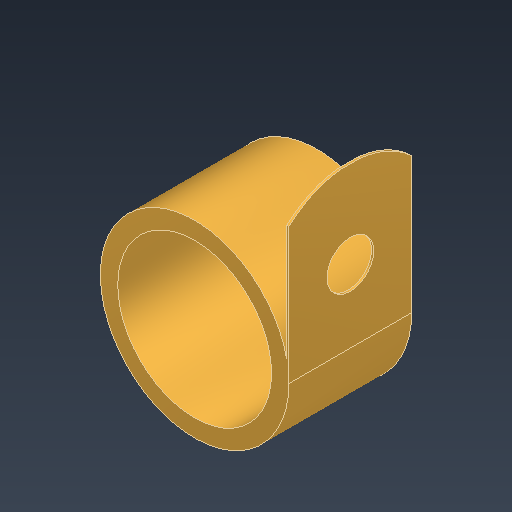
# Autodesk Inventor part: LCF 025 05 031S (on hub)
Saved by Autodesk Inventor 2021.3 (Build 253353000, 353)
## iProperties
Created: 2022-07-28
Part Number: LCF 025 05 031S (on hub)
Material: Brass, Soft Yellow
Document SubType Name: Modeling
Designer: david
Density: 8.47 g/cm^3
Appearance: Brass - Satin
Author: david
Autodesk Inventor part; units mm, degrees
ref_plane "YZ Plane" through (0, 0, 0) normal (1, 0, 0) x (0, 1, 0)
ref_plane "XZ Plane" through (0, 0, 0) normal (0, 1, 0) x (-1, 0, 0)
ref_plane "XY Plane" through (0, 0, 0) normal (0, 0, 1) x (1, 0, 0)
sketch "Sketch1" plane through (0, 0, 0) normal (0, 0, 1) x (1, 0, 0)
  circle A0 centre (0, 0) radius 6.5
  line L0 (6.5, 0) -> (6.35, 0)
  line L1 (6.35, 0) -> (6.35, 11)
  line L2 (6.35, 11) -> (6.5, 11)
  line L3 (6.5, 11) -> (6.5, 0)
  circle A1 centre (0, 0) radius 5.3
  point P0 (6.35, 1.3883)
  dimension "d0" = 13
  dimension "d1" = 0.15
  dimension "d2" = 11
  dimension "d12" = 1.2
  constraints: 8 end point, 2 coincident, 2 parallel, 1 centre point, 1 horizontal, 1 perpendicular, 3 other
  measures "d1" distance of L1.end L2.end
  measures "d2" distance of L2.end L0.start
extrude "Extrusion1" add sketch "Sketch1" along normal blind 8.46
sketch "Sketch2" plane through (6.5, 0, 0) normal (1, 0, 0) x (0, 0, -1)
  circle A0 centre (-4.23, 5) radius 1.61
  line L0 (0, 0) -> (0, 11) projected
  line L1 (-8.46, 0) -> (-8.46, 11) projected
  arc A1 (0, 9.3706) -> (-8.46, 9.3706) centre (-4.23, 4.8377) ccw
  line L2 (-8.46, 0) -> (0, 0)
  line L3 (0, 6.5) -> (0, -6.5) projected
  line L4 (0, 0) -> (0, 11) projected
  line L5 (0, 11) -> (-8.46, 11) projected
  line L6 (-8.46, 0) -> (-8.46, 11) projected
  line L7 (0, 0) -> (-8.46, 0) projected
  point P0 (0, 1.3883)
  point P1 (-3.5473, 11)
  point P2 (-4.9127, 11)
  dimension "d5" = 5
  dimension "d6" = 3.22
  dimension "d8" = 4.23
  dimension "d9" = 6.2
  constraints: 2 centre point, 2 end point, 2 point on circle, 2 point on line, 1 perpendicular
  measures "d5" vertical distance of L0.start A0.centre
  measures "d6" diameter of A0
  measures "d8" distance from line of L0 A0.centre
  measures "d9" radius of A1
extrude "Extrusion2" cut sketch "Sketch2" against normal up to surface (0.15 mm away) contours A0 | A1 L5 L0 | L1 L5 A1
body "Solid1"
